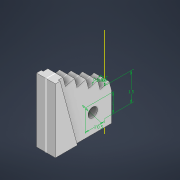
# Autodesk Inventor part: 階梯
Saved by Autodesk Inventor 2021 (Build 250183000, 183)
## iProperties
Created: 2020-12-28
Part Number: 階梯
Material: 一般
Document SubType Name: Modeling
Designer: zihon
Density: 1 g/cm^3
Appearance: 預設
Author: zihon
Autodesk Inventor part; units mm, degrees
ref_plane "YZ Plane" through (0, 0, 0) normal (1, 0, 0) x (0, 1, 0)
ref_plane "XZ Plane" through (0, 0, 0) normal (0, 1, 0) x (-1, 0, 0)
ref_plane "XY Plane" through (0, 0, 0) normal (0, 0, 1) x (1, 0, 0)
sketch "草圖2" plane through (0, 0, 0) normal (1, 0, 0) x (0, 1, 0)
  line L0 (0, 0) -> (1.5, 0)
  line L1 (1.5, 0) -> (1.983, 0.1294)
  line L2 (1.983, 0.1294) -> (1.8536, 0.6124)
  line L3 (1.8536, 0.6124) -> (2.3365, 0.7418)
  line L4 (2.3365, 0.7418) -> (2.2071, 1.2247)
  line L5 (2.2071, 1.2247) -> (2.6901, 1.3542)
  line L6 (2.6901, 1.3542) -> (2.5607, 1.8371)
  line L7 (2.5607, 1.8371) -> (3.0436, 1.9665)
  line L8 (3.0436, 1.9665) -> (2.9142, 2.4495)
  line L9 (2.9142, 2.4495) -> (3.3972, 2.5789)
  line L10 (3.3972, 2.5789) -> (3.3972, 3.0789)
  line L11 (3.3972, 3.0789) -> (0, 3.0789)
  line L12 (0, 3.0789) -> (0, 0)
  circle A0 centre (1, 1) radius 0.25
  line L13 (2.9142, 2.4495) -> (1.5, 0) construction
  line L14 (-0.6794, 0) -> (4.0766, 0) projected
  line L15 (3.3972, 2.5789) -> (2.9142, 2.4495)
  line L16 (3.3972, 2.8289) -> (0, 1.9186)
  point P0 (1.7321, 2.7321)
  dimension "d44" = 1.5
  dimension "d46" = 0.5
  dimension "d48" = 0.5
  dimension "d49" = 15
  dimension "d50" = 0.5
  dimension "d51" = 1
  dimension "d52" = 1
  constraints: 32 end point, 10 perpendicular, 8 equal length, 2 horizontal, 1 centre point, 1 midpoint, 1 parallel, 1 point on line
  measures "d44" distance of L0.start L0.end
  measures "d46" distance of L0.end L1.end
  measures "d48" distance of L1.end L2.end
  measures "d49" angle of L0 L1
  measures "d50" diameter of A0
  measures "d51" horizontal distance of L0.start A0.centre
  measures "d52" horizontal distance of L0.start A0.centre
extrude "擠出1" add sketch "草圖2" along normal mid plane 0.8
extrude "擠出3" add sketch "草圖2" along normal mid plane 1 contours L12 L11 L10 L16
